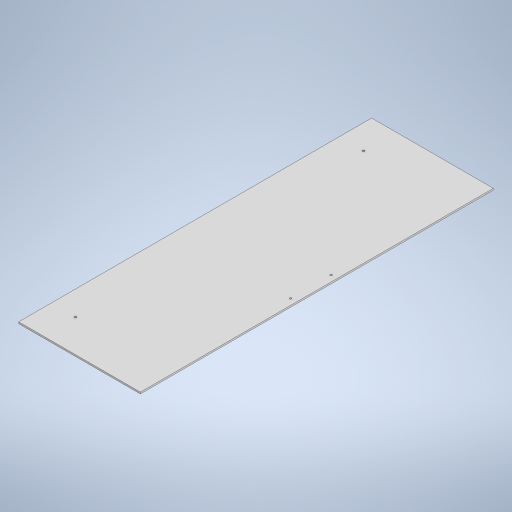
# Autodesk Inventor part: Нижняя полка
Saved by Autodesk Inventor 2023 (Build 270158000, 158)
## iProperties
Created: 2022-05-17
Part Number: Нижняя полка
Material: Типовые
Document SubType Name: Modeling
Designer: avkap
Density: 1 g/cm^3
Appearance: По умолчанию
Author: avkap
Autodesk Inventor part; units mm, degrees
ref_plane "YZ Plane" through (0, 0, 0) normal (1, 0, 0) x (0, 1, 0)
ref_plane "XZ Plane" through (0, 0, 0) normal (0, 1, 0) x (-1, 0, 0)
ref_plane "XY Plane" through (0, 0, 0) normal (0, 0, 1) x (1, 0, 0)
sketch "Эскиз1" plane through (0, 0, 0) normal (0, 1, 0) x (-1, 0, 0)
  line L0 (0, 0) -> (-650, 0)
  line L1 (-650, 0) -> (-650, -870)
  line L2 (-650, -870) -> (0, -870)
  line L3 (0, -870) -> (0, 0)
  line L4 (0, 0) -> (-300, 0)
  line L5 (0, -600) -> (0, 0)
  line L6 (0, -870) -> (-300, -870)
  line L7 (-300, -870) -> (-300, 0)
  line L8 (-300, 0) -> (0, 0)
  line L9 (0, 0) -> (0, -870)
  line L10 (0, 0) -> (-650, -870)
  line L11 (0, -870) -> (-650, 0)
  line L12 (-300, -435) -> (-285, -435)
  line L13 (-285, -435) -> (-285, -385)
  line L14 (-285, -385) -> (-285, -485)
  circle A0 centre (-285, -385) radius 2.5
  circle A1 centre (-285, -485) radius 2.5
  line L15 (0, 0) -> (-59.8526, -80.1104)
  line L16 (0, -870) -> (-59.8526, -789.8896)
  circle A2 centre (-59.8526, -789.8896) radius 2.5
  circle A3 centre (-59.8526, -80.1104) radius 2.5
  dimension "d0" = 650
  dimension "d1" = 870
  dimension "d4" = 15
  dimension "d5" = 50
  dimension "d6" = 100
  dimension "d7" = 5
  dimension "d8" = 5
  dimension "d9" = 100
  dimension "d10" = 100
  dimension "d11" = 5
  dimension "d12" = 5
  constraints: 34 end point, 4 centre point, 4 coincident, 4 horizontal, 4 parallel, 3 perpendicular, 3 point on line, 1 midpoint
  measures "d0" distance of L2.end L1.end
  measures "d1" distance of L1.end L0.end
  measures "d4" distance of L12.start L12.end
  measures "d5" distance of L12.end L13.end
  measures "d6" distance of L13.end L14.end
  measures "d7" diameter of A0
  measures "d8" diameter of A1
  measures "d9" distance of L8.end L15.end
  measures "d10" distance of L2.end L16.end
  measures "d11" diameter of A2
  measures "d12" diameter of A3
extrude "Выдавливание1" add sketch "Эскиз1" along normal blind 4 contours L10 A3 A0 L7 L0 | L3 L11 A2 A1 L14 L13 A0 L10 A3 | L10 A0 L13 L12 L7 | L2 L7 L11 A1 A2 | L12 L14 A1 L11 L7
